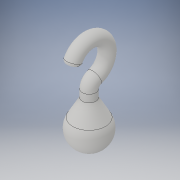
# Autodesk Inventor part: weight hook
Saved by Autodesk Inventor 2019 (Build 230136000, 136)
## iProperties
Created: 2018-09-22
Part Number: weight hook
Material: Generic
Document SubType Name: Modeling
Designer: HIVE
Density: 1 g/cm^3
Appearance: Default
Author: HIVE
Autodesk Inventor part; units mm, degrees
ref_plane "YZ Plane" through (0, 0, 0) normal (1, 0, 0) x (0, 1, 0)
ref_plane "XZ Plane" through (0, 0, 0) normal (0, 1, 0) x (-1, 0, 0)
ref_plane "XY Plane" through (0, 0, 0) normal (0, 0, 1) x (1, 0, 0)
sketch "Sketch1" plane through (0, 0, 0) normal (0, 0, 1) x (1, 0, 0)
  circle A0 centre (0, 0) radius 12.5
  line L0 (0, -12.5) -> (0, 12.5)
  line L1 (0, 12.5) -> (0, 17.5)
  line L2 (0, 17.5) -> (-4.55, 17.5)
  line L3 (-4.55, 17.5) -> (-10.9159, 6.0904)
  dimension "d0" = 25
  dimension "d1" = 5
  constraints: 8 end point, 3 point on circle, 1 centre point, 1 coincident, 1 perpendicular, 1 point on line, 1 tangent, 1 vertical
  measures "d0" diameter of A0
  measures "d1" distance of L0.end L1.end
revolve "Revolution1" add sketch "Sketch1" angle 360 about axis through (0, -12.5, 0) along (0, 1, 0) picked at (-6.02, 0.6319) contours L0 A0 | A0 L3 L2 L1
sketch "Sketch2" plane through (0, 17.5, 0) normal (0, 1, 0) x (1, 0, 0)
  circle A0 centre (0, 0) radius 4.55 projected
sketch "Sketch3" plane through (0, 0, 0) normal (1, 0, 0) x (0, 1, 0)
  arc A0 (27.5204, -3.6628) -> (42.4364, 11.4817) centre (38.9477, 0) ccw
  line L0 (17.5, -4.55) -> (17.5, 4.55) projected
  arc A1 (27.5204, -3.6628) -> (22.5, 0) centre (22.5, -5.272) ccw
  line L1 (17.5, 0) -> (22.5, 0)
  point P0 (0, 0)
  dimension "d3" = 12
  dimension "d4" = 5
  constraints: 4 point on circle, 2 centre point, 2 end point, 2 tangent, 1 horizontal, 1 midpoint, 1 point on line
  measures "d3" radius of A0
  measures "d4" distance of L1.start L1.end
sweep "Sweep1" add profiles "Sketch2" path "Sketch3" path curves L1 A1 A0
fillet "Fillet1" radius 2 1 edges at (-4.55, 42.4364, 11.4817)
body "Solid1"
